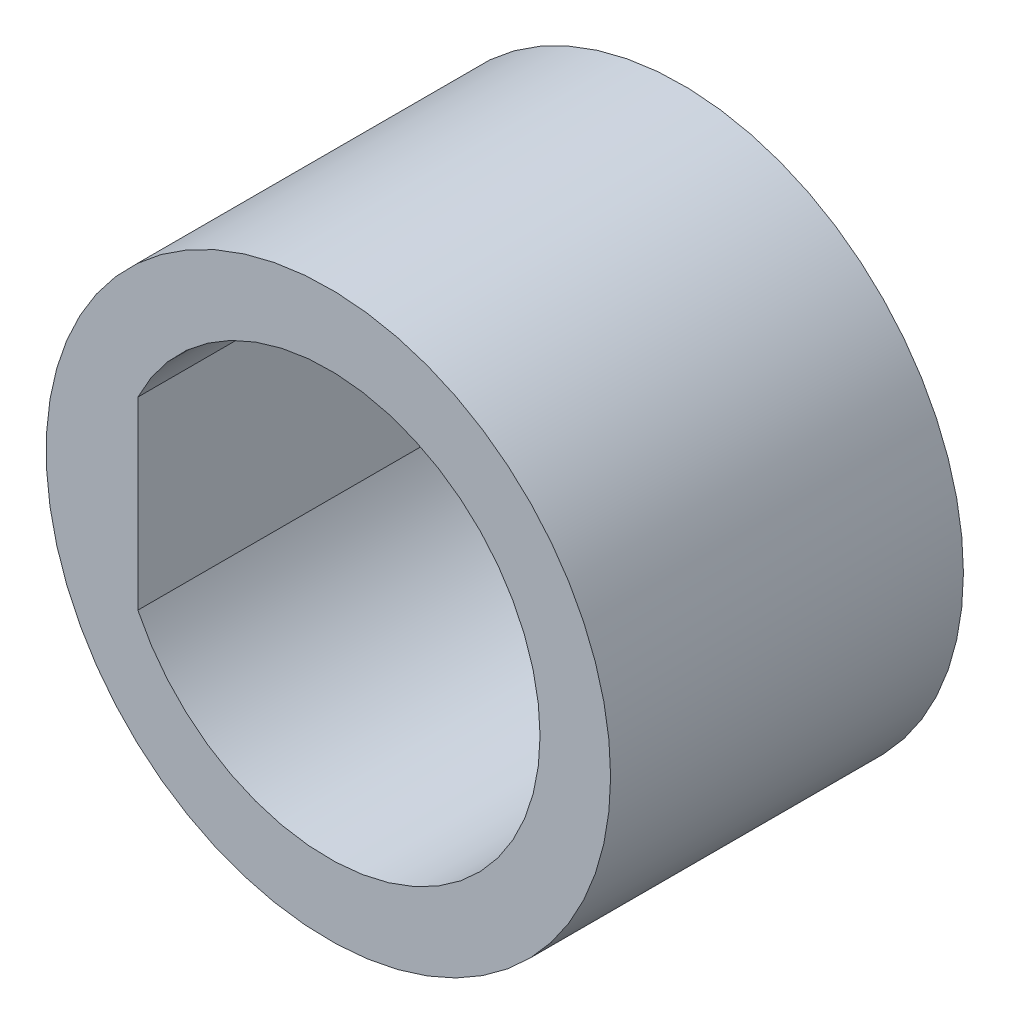
# Autodesk Inventor part: BtnHolder
Saved by Autodesk Inventor 2021 (Build 250183000, 183)
## iProperties
Created: 2021-08-30
Part Number: BtnHolder
Material: Generic
Document SubType Name: Modeling
Designer: teh18
Density: 1 g/cm^3
Appearance: Default
Author: teh18
Autodesk Inventor part; units mm, degrees
ref_plane "YZ Plane" through (0, 0, 0) normal (1, 0, 0) x (0, 1, 0)
ref_plane "XZ Plane" through (0, 0, 0) normal (0, 1, 0) x (-1, 0, 0)
ref_plane "XY Plane" through (0, 0, 0) normal (0, 0, 1) x (1, 0, 0)
ref_plane "Work Plane2" through (0.3, 0, -2) normal (0, 0, 1) x (1, 0, 0)
sketch "Sketch2" plane through (0.3, 0, -2) normal (0, 0, 1) x (1, 0, 0)
  circle A0 centre (-2.8, -2.5) radius 1.1 projected
  circle A1 centre (2.2, -2.5) radius 1.1 projected
  circle A2 centre (-2.8, 2.5) radius 1.1 projected
  circle A3 centre (2.2, 2.5) radius 1.1 projected
  line L0 (-5.7, -2.6153) -> (-5.7, 2.6153) projected
  arc A4 (-5.7, -2.6153) -> (-5.7, 2.6153) centre (-0.3, 0) ccw projected
  circle A5 centre (-0.3, 0) radius 8
  dimension "d2" = 16
  constraints: 1 centre point, 1 coincident
  measures "d2" diameter of A5
extrude "Extrusion1" add sketch "Sketch2" along normal blind 10 contours A5
body "Solid1"
